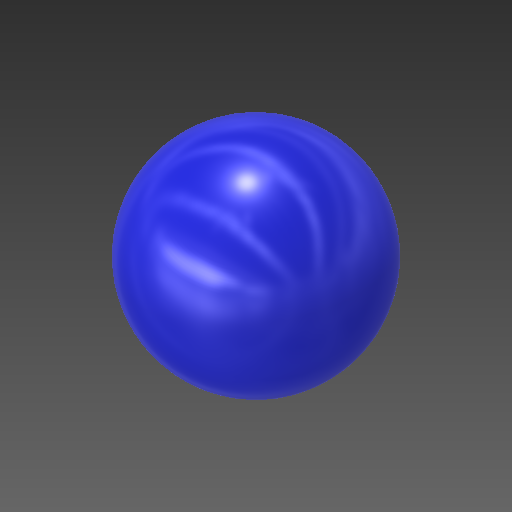
# Autodesk Inventor part: ball
Saved by Autodesk Inventor 2018 (Build 220112000, 112)
## iProperties
Created: 2018-06-15
Part Number: ball
Material: ABS プラスチック
Document SubType Name: Modeling
Designer: NaMACHAN
Density: 1.06 g/cm^3
Appearance: 青 - 壁塗料 - 光沢
Mass: 21.8143 g
Surface Area: 36.3168 cm^2
Volume: 20.5795 cm^3
Author: NaMACHAN
Autodesk Inventor part; units mm, degrees
ref_plane "YZ Plane" through (0, 0, 0) normal (1, 0, 0) x (0, 1, 0)
ref_plane "XZ Plane" through (0, 0, 0) normal (0, 1, 0) x (-1, 0, 0)
ref_plane "XY Plane" through (0, 0, 0) normal (0, 0, 1) x (1, 0, 0)
sketch "スケッチ1" plane through (0, 0, 0) normal (1, 0, 0) x (0, 1, 0)
  arc A0 (17, 0) -> (-17, 0) centre (0, 0) ccw
  line L0 (17, 0) -> (-17, 0)
  point P0 (0, 0)
  dimension "d1" = 17
  constraints: 2 end point, 2 horizontal alignment, 2 point on circle, 1 centre point, 1 horizontal, 1 midpoint, 1 other
  measures "d1" radius of A0
revolve "回転1" add sketch "スケッチ1" angle 360 about axis through (0, 17, 0) along (0, -1, 0)
